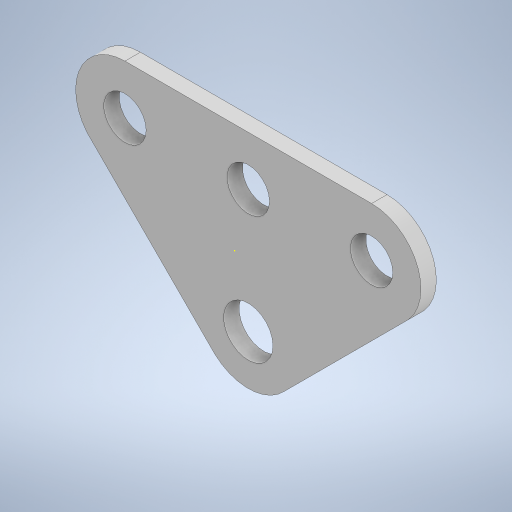
# Autodesk Inventor part: Wing poly connection
Saved by Autodesk Inventor 2023 (Build 270158000, 158)
## iProperties
Created: 2024-01-13
Part Number: Wing poly connection
Material: Generic
Document SubType Name: Modeling
Designer: diego
Density: 1 g/cm^3
Appearance: Default
Author: diego
Autodesk Inventor part; units mm, degrees
ref_plane "YZ Plane" through (0, 0, 0) normal (1, 0, 0) x (0, 1, 0)
ref_plane "XZ Plane" through (0, 0, 0) normal (0, 1, 0) x (-1, 0, 0)
ref_plane "XY Plane" through (0, 0, 0) normal (0, 0, 1) x (1, 0, 0)
sketch "Sketch3" plane through (0, 0, 0) normal (0, 0, 1) x (1, 0, 0)
  circle A0 centre (1.4019, 6.1779) radius 2.1844
  circle A1 centre (-11.2981, 6.1779) radius 2.1844
  circle A2 centre (-23.9981, 6.1779) radius 2.1844
  circle A3 centre (14.1019, 6.1779) radius 2.1844
  line L0 (-11.2981, 6.1779) -> (1.4019, 6.1779)
  line L1 (1.4019, 6.1779) -> (14.1019, 6.1779)
  circle A4 centre (-11.2981, 6.1779) radius 5.08
  circle A5 centre (1.4019, 6.1779) radius 5.08
  circle A6 centre (14.1019, 6.1779) radius 5.08
  line L2 (-11.2981, 11.2579) -> (1.4019, 11.2579)
  line L3 (1.4019, 11.2579) -> (14.1019, 11.2579)
  line L4 (1.4019, 6.1779) -> (1.4019, -6.5221)
  circle A7 centre (1.4019, -6.5221) radius 2.54
  circle A8 centre (1.4019, -6.5221) radius 5.08
  line L5 (-2.0302, -10.2675) -> (-18.1161, 5.8501)
  line L6 (5.1405, -9.9615) -> (17.9077, 2.813)
  point P0 (0, 0)
  point P1 (-15.8845, 3.9935)
  point P2 (18.6882, 3.9935)
  point P3 (4.8339, -10.2675)
  point P4 (-14.5389, 2.2658)
  point P5 (17.3918, 2.2658)
  point P6 (1.4019, -1.4421)
  point P7 (1.4019, 1.0979)
  point P8 (6.4819, 6.1779)
  point P9 (9.0219, 6.1779)
  point P10 (17.4689, 2.374)
  point P11 (-2.3502, -9.9468)
  point P12 (-15.2165, 2.9448)
  point P13 (-3.6781, 6.1779)
  point P14 (-6.2181, 6.1779)
  dimension "d55" = 10.16
  dimension "d54" = 10.16
  dimension "d56" = 10.16
  dimension "d59" = 4.3688
  dimension "d63" = 12.7
  dimension "d64" = 5.08
  dimension "d65" = 10.16
  constraints: 14 end point, 10 point on circle, 8 centre point, 5 coincident, 3 point on line, 2 horizontal, 1 collinear, 3 other
  measures "d54" diameter of A4
  measures "d56" diameter of A6
  measures "d59" diameter of A3
  measures "d63" distance of L4.start L4.end
  measures "d64" diameter of A7
  measures "d65" diameter of A8
extrude "Extrusion7" add sketch "Sketch3" along normal blind 1.5875 contours L1 A5 L4 A0 | A0 L0 A5 L1 | A0 L4 A5 L0 | A5 L3 A6 L1 | L1 A6 L6 A8 L4 A5 | A8 | A5 L4 A8 L5 A4 L0 | L0 A4 L2 A5 | A6 L6 | A4 L5 picked at (18.1676, 5.7732) picked at (-7.2265, 5.798)
sketch "Sketch4" plane through (0, 0, 1.5875) normal (0, 0, 1) x (1, 0, 0)
  point P0 (0, 0)
body "Solid7"
